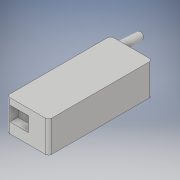
# Autodesk Inventor part: NucPowerBrick
Saved by Autodesk Inventor 2019 (Build 230136000, 136)
## iProperties
Created: 2019-05-22
Part Number: NucPowerBrick
Material: Generic
Document SubType Name: Modeling
Designer: Jorian Bruslind
Density: 1 g/cm^3
Appearance: Default
Author: Jorian Bruslind
Autodesk Inventor part; units mm, degrees
ref_plane "YZ Plane" through (0, 0, 0) normal (1, 0, 0) x (0, 1, 0)
ref_plane "XZ Plane" through (0, 0, 0) normal (0, 1, 0) x (-1, 0, 0)
ref_plane "XY Plane" through (0, 0, 0) normal (0, 0, 1) x (1, 0, 0)
sketch "Sketch1" plane through (0, 0, 0) normal (0, 1, 0) x (-1, 0, 0)
  line L0 (0, 0) -> (52, 0)
  line L1 (52, 0) -> (52, -129)
  line L2 (52, -129) -> (0, -129)
  line L3 (0, -129) -> (0, 0)
  dimension "d0" = 52
  dimension "d1" = 129
  constraints: 8 end point, 2 parallel, 1 horizontal, 1 perpendicular
  measures "d0" distance of L1.end L2.end
  measures "d1" distance of L0.end L1.end
extrude "Extrusion1" add sketch "Sketch1" along normal blind 39
fillet "Fillet1" radius 4 4 edges at (0, 19.5, 0) (0, 19.5, -129) (-52, 19.5, 0) (-52, 19.5, -129)
sketch "Sketch2" plane through (-48, 0, 0) normal (0, 0, 1) x (1, 0, 0)
  line L0 (44, 39) -> (0, 39) projected
  line L1 (0, 39) -> (0, 31)
  line L2 (0, 39) -> (0, 0) projected
  line L3 (0, 31) -> (23, 31)
  line L4 (23, 31) -> (23, 13)
  line L5 (23, 13) -> (0, 13)
  line L6 (0, 13) -> (0, 31)
  point P0 (48, 0)
  dimension "d5" = 8
  dimension "d6" = 23
  dimension "d7" = 18
  constraints: 10 end point, 2 parallel, 1 horizontal, 1 perpendicular, 1 point on line
  measures "d5" distance of L0.end L1.end
  measures "d6" distance of L4.end L5.end
  measures "d7" distance of L3.end L4.end
extrude "Extrusion2" cut sketch "Sketch2" against normal blind 10
sketch "Sketch3" plane through (-4, 0, -129) normal (0, 0, -1) x (-1, 0, 0)
  line L0 (0, 39) -> (44, 39) projected
  line L1 (44, 39) -> (44, 36)
  line L2 (44, 39) -> (44, 0) projected
  line L3 (44, 36) -> (41, 36)
  line L4 (41, 36) -> (36.9695, 31.9695)
  line L5 (41, 36) -> (46.7, 36) construction
  circle A0 centre (36.9695, 31.9695) radius 5.7
  point P0 (-4, 0)
  dimension "d10" = 3
  dimension "d11" = 3
  dimension "d12" = 5.7
  dimension "d13" = 135
  constraints: 8 end point, 1 coincident, 1 equal length, 1 horizontal, 1 perpendicular, 1 point on line, 3 other
  measures "d10" distance of L0.end L1.end
  measures "d11" distance of L1.end L3.end
  measures "d12" distance of L3.end L4.end
  measures "d13" angle of L4 L5
ref_plane "Work Plane1" through (-4, 0, -155) normal (0, 0, -1) x (-1, 0, 0)
sketch "Sketch4" plane through (-4, 0, -155) normal (0, 0, -1) x (-1, 0, 0)
  line L0 (0, 39) -> (44, 39) projected
  line L1 (44, 39) -> (44, 36)
  line L2 (44, 39) -> (44, 0) projected
  line L3 (44, 36) -> (41, 36)
  line L4 (41, 36) -> (36.9695, 31.9695)
  line L5 (41, 36) -> (46.7, 36) construction
  circle A0 centre (36.9695, 31.9695) radius 4.25
  point P0 (-4, 0)
  dimension "d15" = 3
  dimension "d16" = 3
  dimension "d17" = 5.7
  dimension "d18" = 135
  dimension "d19" = 8.5
  constraints: 8 end point, 1 centre point, 1 coincident, 1 equal length, 1 horizontal, 1 perpendicular, 1 point on line
  measures "d15" distance of L0.end L1.end
  measures "d16" distance of L1.end L3.end
  measures "d17" distance of L3.end L4.end
  measures "d18" angle of L4 L5
  measures "d19" diameter of A0
loft "Loft1" add profiles "Sketch3", "Sketch4"
body "Solid1"
